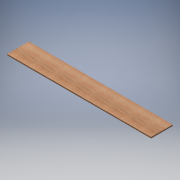
# Autodesk Inventor part: estante02
Saved by Autodesk Inventor 2016 (Build 200138000, 138)
## iProperties
Created: 2018-06-25
Part Number: estante02
Material: Wood (Birch)
Document SubType Name: Modeling
Designer: damia
Density: 0.55 g/cm^3
Appearance: Birch - Natural Polished
Mass: 5940 g
Surface Area: 12828 cm^2
Volume: 10800 cm^3
Author: damia
Autodesk Inventor part; units mm, degrees
ref_plane "YZ Plane" through (0, 0, 0) normal (1, 0, 0) x (0, 1, 0)
ref_plane "XZ Plane" through (0, 0, 0) normal (0, 1, 0) x (-1, 0, 0)
ref_plane "XY Plane" through (0, 0, 0) normal (0, 0, 1) x (1, 0, 0)
sketch "Sketch1" plane through (0, 0, 0) normal (0, 0, 1) x (1, 0, 0)
  line L0 (1975, 75) -> (1075, 75) projected
  line L1 (1075, 75) -> (1075, -225) projected
  line L2 (1075, -225) -> (1975, -225) projected
  line L3 (1975, -225) -> (1975, 75) projected
  line L4 (1975, -225) -> (-25, -225)
  line L5 (-25, -225) -> (-25, 75)
  line L6 (-25, 75) -> (1975, 75)
  line L7 (1975, 75) -> (1975, -225)
  point P0 (0, 0)
  dimension "d0" = 25
  constraints: 8 end point, 2 parallel, 1 horizontal, 1 perpendicular
  measures "d0" distance from line of L5 point (0, 0)
extrude "Extrusion1" add sketch "Sketch1" along normal blind 18
body "Solid1"
